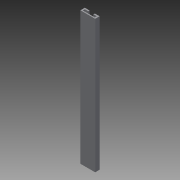
# Autodesk Inventor part: Channel II
Saved by Autodesk Inventor 2014 (Build 180170000, 170)
## iProperties
Created: 2014-07-22
Part Number: Channel II
Material: Generic
Document SubType Name: Modeling
Designer: quinn
Density: 1 g/cm^3
Appearance: Default
Author: quinn
Autodesk Inventor part; units mm, degrees
ref_plane "YZ Plane" through (0, 0, 0) normal (1, 0, 0) x (0, 1, 0)
ref_plane "XZ Plane" through (0, 0, 0) normal (0, 1, 0) x (-1, 0, 0)
ref_plane "XY Plane" through (0, 0, 0) normal (0, 0, 1) x (1, 0, 0)
sketch "Sketch1" plane through (0, 0, 0) normal (0, 1, 0) x (-1, 0, 0)
  line L0 (-19.3426, 10.7847) -> (6.0574, 10.7847)
  line L1 (6.0574, 10.7847) -> (6.0574, 3.1647)
  line L2 (-19.3426, 3.1647) -> (-19.3426, 10.7847)
  line L3 (-2.1341, 3.1647) -> (-2.1341, 5.5142)
  line L4 (-11.1511, 5.5142) -> (-11.1511, 3.1647)
  line L5 (-16.8661, 8.9432) -> (3.5809, 8.9432)
  line L6 (3.5809, 8.9432) -> (3.5809, 5.5142)
  line L7 (-16.8661, 5.5142) -> (-16.8661, 8.9432)
  line L8 (3.5809, 5.5142) -> (-2.1341, 5.5142)
  line L9 (-11.1511, 5.5142) -> (-16.8661, 5.5142)
  line L10 (6.1209, 3.1647) -> (-2.1341, 3.1647)
  line L11 (-11.1511, 3.1647) -> (-19.4061, 3.1647)
  line L12 (6.0574, 3.1647) -> (-2.1341, 3.1647)
  line L13 (-11.1511, 3.1647) -> (-19.3426, 3.1647)
  point P0 (0, 0)
  point P1 (0, 0)
  dimension "d0" = 7.62
  dimension "d1" = 8.1915
  dimension "d2" = 8.1915
  dimension "d3" = 25.4
  dimension "d4" = 2.3495
  dimension "d5" = 2.3495
  dimension "d6" = 5.715
  dimension "d7" = 5.715
  dimension "d8" = 3.429
  constraints: 28 end point, 7 parallel, 2 horizontal, 2 perpendicular
  measures "d0" distance of L0.end L1.end
  measures "d1" distance of L1.end L3.start
  measures "d2" distance of L4.end L13.end
  measures "d3" distance between parallel lines of L1 L2
  measures "d4" distance of L3.start L3.end
  measures "d5" distance of L4.start L4.end
  measures "d6" distance of L8.start L3.end
  measures "d7" distance of L4.start L9.end
  measures "d8" distance of L9.end L5.start
extrude "Extrusion1" add sketch "Sketch1" along normal blind 228.6
body "Solid1"
